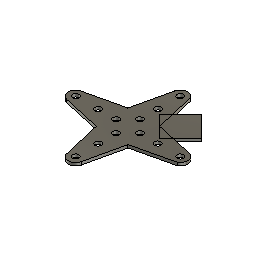
Drone Motor Mount v1 (Autodesk Fusion 360 design; units mm, degrees)
Autodesk Fusion 360 part; units mm, degrees
sketch "Frame" plane through (0, 0, 0) normal (0, 0, 1) x (1, 0, 0)
  circle A0 centre (0, 0) radius 35 construction
  circle A1 centre (0, 0) radius 8 construction
  line L0 (0, 0) -> (0, 2.9787)
  line L1 (0, 2.9787) -> (0, 35) construction
  circle A2 centre (0, 8) radius 2.1
  circle A3 centre (0, 0) radius 11 construction
  circle A4 centre (0, 0) radius 20 construction
  circle A5 centre (0, 35) radius 2.1
  circle A6 centre (0, 20) radius 2.1
  circle A7 centre (0, 35) radius 5
  line L2 (0, 0) -> (24.7487, 24.7487) construction
  line L3 (0, 0) -> (35, 0) construction
  line L4 (0, 21.2132) -> (-21.2132, 0) construction
  line L5 (-21.2132, 0) -> (0, -21.2132) construction
  line L6 (0, -21.2132) -> (21.2132, 0) construction
  line L7 (21.2132, 0) -> (0, 21.2132) construction
  line L8 (-4.8965, 36.0123) -> (-10.6066, 10.6066)
  line L9 (4.354, 37.4581) -> (10.6066, 10.6066)
  line L10 (-37.4581, 4.354) -> (-10.6066, 10.6066)
  line L11 (-36.0123, -4.8965) -> (-10.6066, -10.6066)
  circle A8 centre (-35, 0) radius 5
  circle A9 centre (-35, 0) radius 2.1
  circle A10 centre (-20, 0) radius 2.1
  circle A11 centre (-8, 0) radius 2.1
  line L12 (-4.354, -37.4581) -> (-10.6066, -10.6066)
  line L13 (4.8965, -36.0123) -> (10.6066, -10.6066)
  circle A12 centre (0, -35) radius 5
  circle A13 centre (0, -35) radius 2.1
  circle A14 centre (0, -20) radius 2.1
  circle A15 centre (0, -8) radius 2.1
  line L14 (37.4581, -4.354) -> (10.6066, -10.6066)
  line L15 (36.0123, 4.8965) -> (10.6066, 10.6066)
  circle A16 centre (35, 0) radius 5
  circle A17 centre (35, 0) radius 2.1
  circle A18 centre (20, 0) radius 2.1
  circle A19 centre (8, 0) radius 2.1
  dimension "d1" = 70
  dimension "d2" = 16
  dimension "d3" = 4.2
  dimension "d4" = 22
  dimension "d5" = 40
  dimension "d6" = 4.2
  dimension "d7" = 4.2
  dimension "d8" = 10
  dimension "d10" = 45
  dimension "d11" = 15
  dimension "d13" = 360
  constraint coincident A0.centre A1.centre
  constraint concentric A0 A1
  constraint vertical L0
  constraint coincident A0 L1.end
  constraint parallel L0 L1
  constraint coincident L1 A2.centre
  constraint coincident A1 A2.centre
  constraint concentric A0 A3
  constraint concentric A0 A4
  constraint coincident L1.end A5.centre
  constraint coincident L1 A6.centre
  constraint coincident A4 A6.centre
  constraint concentric A5 A7
  constraint horizontal L3
  constraint coincident A7 L8.start
  constraint midpoint L4 L8.end
  constraint coincident A7 L9.start
  constraint midpoint L7 L9.end
  measures "d1" diameter of A0
  measures "d2" diameter of A1
  measures "d3" diameter of A2
  measures "d4" diameter of A3
  measures "d5" diameter of A4
  measures "d6" diameter of A5
  measures "d7" diameter of A6
  measures "d8" diameter of A7
  measures "d10" angle of L2 L3
  measures "d11" distance of A0.centre L7
sketch "Wire Rest" plane through (0, 0, 0) normal (0, 0, 1) x (1, 0, 0)
  line L0 (21.2132, 0) -> (0, 21.2132)
  line L1 (10.6066, 10.6066) -> (3.5355, 17.6777)
  line L2 (10.6066, 10.6066) -> (17.6777, 3.5355)
  line L3 (3.5355, 17.6777) -> (17.6777, 31.8198)
  line L4 (17.6777, 3.5355) -> (31.8198, 17.6777)
  line L5 (17.6777, 31.8198) -> (31.8198, 17.6777)
  dimension "d14" = 10
  dimension "d15" = 10
  dimension "d16" = 20
  dimension "d18" = 20
  constraint midpoint L0 L1.start
  constraint coincident L0 L1.end
  constraint parallel L0 L2
  constraint perpendicular L1 L3
  constraint perpendicular L2 L4
  measures "d14" distance of L1.start L1.end
  measures "d15" distance of L1.start L2.end
  measures "d16" distance of L1.end L3.end
  measures "d18" distance of L2.end L4.end
extrude "Extrude1" add sketch "Frame" along normal blind 2 contours A7 L9 | A7 L8 L9 L10 L11 A8 L12 L13 A12 L14 L15 A16 | L14 A16 | L10 A8 | L12 A12 picked at (3.7843, 35.9318) picked at (35.8812, -3.7978) picked at (-35.8812, 3.7978) picked at (-3.7843, -35.9318) makes body 1
extrude "Extrude2" add sketch "Wire Rest" along normal blind 2 separate body makes body 2
